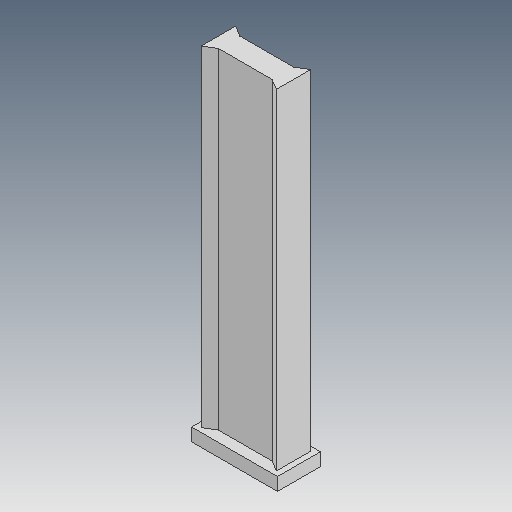
# Autodesk Inventor part: drawerconnector
Saved by Autodesk Inventor 2025.2 (Build 292293000, 293)
## iProperties
Created: 2025-02-24
Part Number: drawerconnector
Material: Generic
Document SubType Name: Modeling
Designer: email
Density: 1 g/cm^3
Appearance: Default
Author: email
Autodesk Inventor part; units mm, degrees
ref_plane "YZ Plane" through (0, 0, 0) normal (1, 0, 0) x (0, 1, 0)
ref_plane "XZ Plane" through (0, 0, 0) normal (0, 1, 0) x (-1, 0, 0)
ref_plane "XY Plane" through (0, 0, 0) normal (0, 0, 1) x (1, 0, 0)
sketch "Sketch1" plane through (0, 0, 0) normal (0, 1, 0) x (-1, 0, 0)
  line L0 (0, -2.5) -> (-6.25, -2.5)
  line L1 (-6.25, -2.5) -> (-8.75, -4)
  line L2 (-8.75, -4) -> (-8.75, 4)
  line L3 (-8.75, 4) -> (-6.25, 2.5)
  line L4 (-6.25, 2.5) -> (0, 2.5)
  line L5 (0, 2.5) -> (0, -2.5)
  line L6 (0, -5) -> (-10, -5)
  line L7 (-10, -5) -> (-10, 5)
  line L8 (-10, 5) -> (0, 5)
  line L9 (0, 5) -> (0, -5)
  point P0 (-8.75, 0)
  point P1 (0, 0)
  point P2 (0, 0)
  point P3 (0, 2.5)
  dimension "d16" = 5
  dimension "d17" = 2.5
  dimension "d18" = 8
  dimension "d19" = 8.75
  dimension "d20" = 10
  dimension "d21" = 5
  dimension "d22" = 5
  constraints: 20 end point, 3 parallel, 3 perpendicular, 2 horizontal, 2 midpoint, 1 coincident, 1 horizontal alignment, 1 vertical alignment
  measures "d16" distance of L3.end L0.end
  measures "d17" distance from line of L2 L0.end
  measures "d18" distance of L1.end L2.end
  measures "d19" distance between parallel lines of L5 L2
  measures "d20" distance between parallel lines of L9 L7
  measures "d21" distance from line of point (0, 0) L6
  measures "d22" distance from line of point (0, 0) L8
extrude "Extrusion1" add sketch "Sketch1" along normal blind 3
extrude "Extrusion2" add sketch "Sketch1" along normal blind 80 contours L0 L1 L2 L3 L4 L5
mirror "Mirror1" about plane through (0, 0, -5) normal (-1, 0, 0) of "Extrusion1", "Extrusion2"
body "Solid1"
